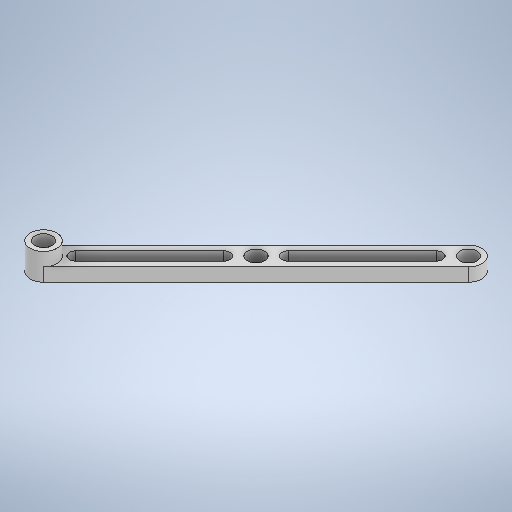
# Autodesk Inventor part: Bump Arm
Saved by Autodesk Inventor 2025.1 (Build 291241000, 241)
## iProperties
Created: 2025-10-25
Part Number: Bump Arm
Material: Generic
Document SubType Name: Modeling
Designer: benja
Density: 1 g/cm^3
Appearance: Default
Author: benja
Autodesk Inventor part; units mm, degrees
ref_plane "YZ Plane" through (0, 0, 0) normal (1, 0, 0) x (0, 1, 0)
ref_plane "XZ Plane" through (0, 0, 0) normal (0, 1, 0) x (-1, 0, 0)
ref_plane "XY Plane" through (0, 0, 0) normal (0, 0, 1) x (1, 0, 0)
sketch "Sketch1" plane through (0, 0, 0) normal (0, 1, 0) x (-1, 0, 0)
  circle A0 centre (-56.7045, -56.3864) radius 4.8895
  circle A1 centre (-56.7045, -56.3864) radius 4.8895
  line L0 (-52.2143, -60.8765) -> (69.7375, 61.0754)
  line L1 (60.7573, 70.0556) -> (-61.1946, -51.8963)
  arc A2 (-61.1946, -51.8963) -> (-52.2143, -60.8765) centre (-56.7045, -56.3864) ccw
  arc A3 (69.7375, 61.0754) -> (60.7573, 70.0556) centre (65.2474, 65.5655) ccw
  circle A4 centre (4.2715, 4.5895) radius 4.8895
  circle A5 centre (65.2474, 65.5655) radius 4.8895
  line L2 (7.7289, 8.0469) -> (61.79, 62.1081)
  line L3 (68.7048, 69.0229) -> (69.7375, 70.0556)
  line L4 (-53.2471, -52.929) -> (0.8141, 1.1322) construction
  line L5 (7.7289, 8.0469) -> (61.79, 62.1081) construction
  line L6 (0.8141, 1.1322) -> (-53.2471, -52.929)
  line L7 (-60.1619, -59.8438) -> (-61.1946, -60.8765)
  line L8 (-5.0037, -4.6857) -> (-47.4293, -47.1112) construction
  line L9 (-7.5546, -2.1348) -> (-49.9802, -44.5603)
  line L10 (-44.8784, -49.6621) -> (-2.4529, -7.2365)
  arc A6 (-2.4529, -7.2365) -> (-7.5546, -2.1348) centre (-5.0037, -4.6857) ccw
  arc A7 (-49.9802, -44.5603) -> (-44.8784, -49.6621) centre (-47.4293, -47.1112) ccw
  line L11 (4.2715, 4.5895) -> (-0.2187, 9.0797)
  arc A8 (10.9958, 16.4156) -> (16.0976, 11.3139) centre (13.5467, 13.8648) ccw
  line L12 (10.9958, 16.4156) -> (53.4213, 58.8412)
  line L13 (58.5231, 53.7394) -> (16.0976, 11.3139)
  arc A9 (58.5231, 53.7394) -> (53.4213, 58.8412) centre (55.9722, 56.2903) ccw
  line L14 (70.6356, 60.1773) -> (-51.3163, -61.7745)
  arc A10 (-62.0926, -50.9982) -> (-51.3163, -61.7745) centre (-56.7045, -56.3864) ccw
  line L15 (-62.0926, -50.9982) -> (59.8592, 70.9536)
  arc A11 (70.6356, 60.1773) -> (59.8592, 70.9536) centre (65.2474, 65.5655) ccw
  circle A12 centre (65.2474, 65.5655) radius 7.62
  point P0 (0, 0)
  point P1 (29.6663, 4.6577)
  point P2 (-26.2165, -25.8984)
  dimension "d0" = 172.466
  dimension "d1" = 12.7
  dimension "d2" = 9.779
  dimension "d3" = 9.779
  dimension "d4" = 9.779
  dimension "d9" = 1.27
  constraints: 34 end point, 24 point on circle, 13 centre point, 8 tangent, 6 symmetric about line, 3 coincident, 3 midpoint, 3 parallel, 1 concentric, 1 point on line, 5 other
  measures "d0" distance of A1.centre A3.centre
  measures "d1" diameter of A3
  measures "d2" diameter of A4
  measures "d3" diameter of A1
  measures "d4" diameter of A5
  measures "d9" distance between parallel lines of L0 L14
extrude "Extrusion1" add sketch "Sketch1" along normal blind 7.62 contours A0 L6 A7 L10 A6 A4 L2 A8 L13 A9 A12 L0 A2 L7 | A0 L7 A2 L1 L11 A4 L6 A6 L9 A7 | L1 A12 L2 A9 L12 A8 A4 L11 | A12 L2 A5 L3 A3 L0 | L1 A3 L3 A5 L2 A12
sketch "Sketch2" plane through (0, 7.62, 0) normal (0, 1, 0) x (1, 0, 0)
  line L0 (-60.7573, -70.0556) -> (61.1946, 51.8963) projected
  arc A0 (61.1946, 51.8963) -> (52.2143, 60.8765) centre (56.7045, 56.3864) ccw projected
  line L1 (52.2143, 60.8765) -> (-69.7375, -61.0754) projected
  arc A1 (-69.7375, -61.0754) -> (-60.7573, -70.0556) centre (-65.2474, -65.5655) ccw projected
  arc A2 (-58.5231, -53.7394) -> (-53.4213, -58.8412) centre (-55.9722, -56.2903) ccw projected
  line L2 (-58.5231, -53.7394) -> (-16.0976, -11.3139) projected
  arc A3 (-10.9958, -16.4156) -> (-16.0976, -11.3139) centre (-13.5467, -13.8648) ccw projected
  line L3 (-10.9958, -16.4156) -> (-53.4213, -58.8412) projected
  circle A4 centre (-65.2474, -65.5655) radius 4.8895 projected
  circle A5 centre (-4.2715, -4.5895) radius 4.8895 projected
  circle A6 centre (56.7045, 56.3864) radius 4.8895 projected
  arc A7 (49.9802, 44.5603) -> (44.8784, 49.6621) centre (47.4293, 47.1112) ccw projected
  line L4 (49.9802, 44.5603) -> (7.5546, 2.1348) projected
  arc A8 (2.4529, 7.2365) -> (7.5546, 2.1348) centre (5.0037, 4.6857) ccw projected
  line L5 (2.4529, 7.2365) -> (44.8784, 49.6621) projected
  circle A9 centre (-65.2474, -65.5655) radius 6.35
  point P0 (0, 0)
  constraints: 1 centre point, 1 coincident, 1 tangent
extrude "Extrusion2" add sketch "Sketch2" along normal blind 7.62 contours A1 A9
extrude "Extrusion3" add sketch "Sketch1" along normal blind 7.62 contours A2 L0 A12 L14 A10 L15 L1 | L0 A3 L1 A12 A11
extrude "Extrusion4" add sketch "Sketch1" along normal up to surface (15.24 mm away) contours A12 L2 A5 L3 A3 L0 | L0 A3 L1 A12 A11 | L1 A3 L3 A5 L2 A12 | A5
extrude "Extrusion5" cut sketch "Sketch1" along normal blind 25.4 contours A5
body "Solid1"
